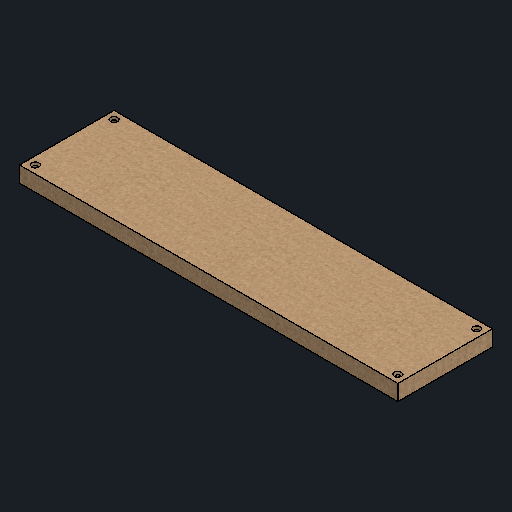
# Autodesk Inventor part: Part3
Saved by Autodesk Inventor 2026.2 (Build 302298000, 298)
## iProperties
Created: 2026-06-15
Part Number: Part3
Material: MDF Medium Density Fiberboard
Document SubType Name: Modeling
Designer: JoshuaEah
Density: 0.8 g/cm^3
Appearance: Cardboard - Corrugated
Author: JoshuaEah
Autodesk Inventor part; units mm, degrees
ref_plane "YZ Plane" through (0, 0, 0) normal (1, 0, 0) x (0, 1, 0)
ref_plane "XZ Plane" through (0, 0, 0) normal (0, 1, 0) x (-1, 0, 0)
ref_plane "XY Plane" through (0, 0, 0) normal (0, 0, 1) x (1, 0, 0)
sketch "Sketch1" plane through (0, 0, 0) normal (0, 1, 0) x (-1, 0, 0)
  line L0 (0, 0) -> (-304.8, 0)
  line L1 (-304.8, 0) -> (-304.8, -76.2)
  line L2 (-304.8, -76.2) -> (0, -76.2)
  line L3 (0, -76.2) -> (0, 0)
  circle A0 centre (-6.35, -69.85) radius 1.3891
  circle A1 centre (-6.35, -6.35) radius 1.3891
  circle A2 centre (-298.45, -6.35) radius 1.3891
  circle A3 centre (-298.45, -69.85) radius 1.3891
  dimension "d0" = 76.2
  dimension "d1" = 304.8
  dimension "d4" = 2.7781
  dimension "d5" = 6.35
  dimension "d6" = 6.35
  dimension "d7" = 6.35
  dimension "d8" = 6.35
  constraints: 8 end point, 4 centre point, 3 equal radius, 2 horizontal alignment, 2 parallel, 2 vertical alignment, 1 coincident, 1 horizontal, 1 perpendicular
  measures "d0" distance of L2.end L0.start
  measures "d1" distance of L0.start L0.end
  measures "d4" diameter of A0
  measures "d5" distance from line of A0.centre L3
  measures "d6" distance from line of L2 A0.centre
  measures "d7" distance from line of L1 A3.centre
  measures "d8" distance from line of L0 A1.centre
extrude "Extrusion1" add sketch "Sketch1" against normal blind 12.7 contours L3 L2 L1 L0 | A0 | A1 | A2 | A3
hole "Hole1" at (6.35, 0, -69.85) at (298.45, 0, -69.85) at (298.45, 0, -6.35) at (6.35, 0, -6.35) direction (0, -1, 0) diameter 3.2766 end through all countersink diameter 5.715 countersink angle 82 clearance for "Flat Head Machine Screw (82)" size "#4" standard "Ansi Unified Screw Threads"
equation "\"d7\" = d5"
equation "\"d8\" = d6"
body "Solid1"
